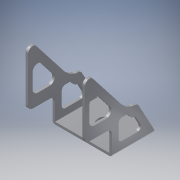
# Autodesk Inventor part: 頭_メインフレーム_1_1
Saved by Autodesk Inventor 2018 (Build 220112000, 112)
## iProperties
Created: 2016-05-10
Part Number: 頭_メインフレーム_1_1
Material: アルミニウム 5052
Document SubType Name: シート メタル
Designer: hiroaki
Density: 2.68 g/cm^3
Sheet Metal Rule: Default_mm
Appearance: アルミニウム - フラット
Mass: 7.8172 g
Surface Area: 48.1184 cm^2
Volume: 2.91687 cm^3
Flat Pattern Width: 4.175 cm
Flat Pattern Length: 12.6574 cm
Flat Pattern Area: 52.8444 cm^2
Sheet Metal Width: 41.750 mm
Sheet Metal Length: 126.574 mm
Sheet Metal Area: 5284.444 mm^2
Author: hiroaki
Autodesk Inventor part; units mm, degrees
ref_plane "YZ Plane" through (0, 0, 0) normal (1, 0, 0) x (0, 1, 0)
ref_plane "XZ Plane" through (0, 0, 0) normal (0, 1, 0) x (-1, 0, 0)
ref_plane "XY Plane" through (0, 0, 0) normal (0, 0, 1) x (1, 0, 0)
sketch "スケッチ1" plane through (0, 0, 0) normal (0, 0, 1) x (1, 0, 0)
  circle A0 centre (0, 0) radius 11 construction
  circle A1 centre (0, 8.5) radius 1.35
  circle A2 centre (0, 0) radius 5.05
  circle A3 centre (-8.5, 0) radius 1.35
  circle A4 centre (0, -8.5) radius 1.35
  circle A5 centre (8.5, 0) radius 1.35
  line L0 (-16.25, 11) -> (-16.25, -30.75)
  line L1 (-16.25, -30.75) -> (16.25, -30.75)
  line L2 (16.25, -30.75) -> (16.25, 11)
  line L3 (16.25, 11) -> (-16.25, 11)
  line L4 (-13.5, -1) -> (13.5, -1) construction
  line L5 (13.5, -1) -> (13.5, -28) construction
  line L6 (13.5, -28) -> (-13.5, -28) construction
  line L7 (-13.5, -28) -> (-13.5, -1) construction
  circle A6 centre (-13.5, -1) radius 1.35 construction
  circle A7 centre (-13.5, -1) radius 2.75 construction
  circle A8 centre (-13.5, -28) radius 2.75 construction
  point P0 (0, 11)
  point P1 (0, -30.75)
  point P2 (0, -1)
  dimension "d0" = 22
  dimension "d1" = 10.1
  dimension "d2" = 8.5
  dimension "d3" = 2.7
  dimension "d6" = 360
  dimension "d8" = 32.5
  dimension "d9" = 27
  dimension "d10" = 1
  dimension "d11" = 2.7
  dimension "d40" = 41.75
  constraints: 16 end point, 9 centre point, 5 coincident, 4 perpendicular, 4 tangent, 4 vertical alignment, 3 midpoint, 3 parallel, 1 horizontal, 1 vertical, 9 other
  measures "d0" diameter of A0
  measures "d1" diameter of A2
  measures "d2" distance of point (0, 0) A1.centre
  measures "d3" diameter of A1
  measures "d8" distance between parallel lines of L2 L0
  measures "d9" distance of L4.start L4.end
  measures "d10" distance from line of point (0, 0) L4
  measures "d11" diameter of A6
  measures "d40" distance between parallel lines of L3 L1
extrude "押し出し1" add sketch "スケッチ1" along normal blind 1.5
sketch "スケッチ2" plane through (-16.25, -30.75, 1.5001) normal (-1, 0, 0) x (0, -1, 0)
  line L0 (-41.75, 0) -> (0, 0)
  line L1 (0, 0) -> (0, 45.9999)
  line L2 (0, 45.9999) -> (-41.75, 45.9999)
  line L3 (-41.75, 45.9999) -> (-41.75, 0)
  constraints: 6 end point, 1 horizontal, 1 perpendicular, 1 vertical
edge flange "フランジ1" height 47.5 angle 90 thickness 1.5 bend radius 0.0001 thickness toward (-1, 0, 0) relief straight relief width 1.5 relief depth 0.75 edges at (-16.25, -9.875, 1.5) wall of the first edge with corners at (-16.25, 11, 1.5001) (-16.25, -30.75, 1.5001) (-16.2501, -30.75, 47.5) (-16.2501, 11, 47.5)
bend "曲げ1"
corner "コーナー1"
sketch "スケッチ3" plane through (-17.75, -30.75, 47.5) normal (-1, 0, 0) x (0, 0, 1)
  line L0 (0, 41.75) -> (0, 0) projected
  line L1 (-45.9999, 41.75) -> (0, 41.75) projected
  line L2 (-2.75, 29.75) -> (-29.75, 29.75) construction
  line L3 (-29.75, 29.75) -> (-29.75, 2.75) construction
  line L4 (-29.75, 2.75) -> (-2.75, 2.75) construction
  line L5 (-2.75, 2.75) -> (-2.75, 29.75) construction
  line L6 (0, 0) -> (-45.9999, 0) construction
  circle A0 centre (-2.75, 29.75) radius 1.35
  circle A1 centre (-2.75, 2.75) radius 1.35
  circle A2 centre (-29.75, 2.75) radius 1.35
  circle A3 centre (-29.75, 29.75) radius 1.35
  circle A4 centre (-2.75, 2.75) radius 2.75 construction
  line L7 (-23.0232, 22.0826) -> (-1.0567, 4.9169)
  arc A5 (-2.75, 0) -> (-1.0567, 4.9169) centre (-2.75, 2.75) ccw
  line L8 (-2.75, 0) -> (-2.75, -11.4677)
  line L9 (-2.75, -11.4677) -> (6.4192, -11.4677)
  line L10 (6.4192, -11.4677) -> (6.4192, 48.6525)
  line L11 (6.4192, 48.6525) -> (-30.25, 50.6687)
  circle A6 centre (-29.75, 29.75) radius 2.75 construction
  circle A7 centre (-16.25, 30.75) radius 11 construction
  arc A8 (-27.2491, 30.8936) -> (-23.0232, 22.0826) centre (-16.25, 30.75) ccw
  line L12 (-5.4497, 3.2733) -> (-25.4861, 18.9308)
  arc A9 (-5.4497, 3.2733) -> (-5.5, 2.75) centre (-2.75, 2.75) ccw
  arc A10 (-25.75, 19.1418) -> (-25.4861, 18.9308) centre (-16.25, 30.75) ccw
  line L13 (-5.5, 2.75) -> (-25.75, 2.75)
  line L14 (-25.75, 2.75) -> (-25.75, 19.1418)
  arc A11 (-27.2491, 30.8936) -> (-28.4327, 32.164) centre (-29.75, 29.75) ccw
  line L15 (-28.4327, 32.164) -> (-45.9999, 41.75)
  line L16 (-45.9999, 41.75) -> (-30.25, 50.6687)
  point P0 (-47.5, 30.75)
  point P1 (-2.75, 16.25)
  point P2 (-16.25, 29.75)
  dimension "d24" = 27
  dimension "d30" = 2.7
  dimension "d44" = 12
  dimension "d45" = 1
  dimension "d46" = 22
  dimension "d50" = 4
  dimension "d52" = 4
  constraints: 28 end point, 11 centre point, 11 coincident, 10 point on circle, 5 tangent, 4 perpendicular, 3 concentric, 3 equal radius, 3 parallel, 2 horizontal, 2 midpoint, 2 vertical, 2 vertical alignment, 1 collinear, 6 other
  measures "d24" distance of L2.start L2.end
  measures "d30" diameter of A0
  measures "d44" distance between parallel lines of L1 L2
  measures "d45" distance from line of L2 A7.centre
  measures "d46" diameter of A7
  measures "d50" radial gap between concentric circles of A10 A8
  measures "d52" distance between parallel lines of L3 L14
extrude "押し出し2" cut sketch "スケッチ3" against normal blind 1.5 contours L1 L16 L11 L10 L9 L8 A5 L0 | L0 A5 L7 A8 A11 L15 L1 | A0 | A1 | A2 | A3 | A9 L13 L14 A10 L12
mirror "ミラー1" about plane through (0, 0, 0) normal (1, 0, 0) of "押し出し2", "フランジ1"
sketch "スケッチ5" plane through (-17.75, -30.75, 1.5001) normal (-1, 0, 0) x (0, 0, 1)
  circle A0 centre (16.25, 2.75) radius 1.35 projected
  line L0 (43.25, 0) -> (0, 0) projected
  line L1 (-3.1343, -10.7624) -> (13.5, -10.7624)
  line L2 (13.5, -10.7624) -> (13.5, 16.25)
  line L3 (13.5, 16.25) -> (-3.1343, 16.25)
  line L4 (-3.1343, 16.25) -> (-3.1343, -10.7624)
  circle A1 centre (16.25, 2.75) radius 2.75 construction
  point P0 (-1.5, 30.75)
  dimension "d47" = 13.5
  constraints: 8 end point, 2 parallel, 2 tangent, 1 centre point, 1 coincident, 1 horizontal, 1 perpendicular
  measures "d47" distance from line of A0.centre L3
extrude "押し出し4" cut sketch "スケッチ5" against normal blind 100 contours L4 L3 L2 L1
fillet "フィレット1" radius 3 6 edges at (17, 0.1436, 20.2509) (-17, 0.1436, 20.2509) (-17, -14.5, 15) (-17, -30.75, 15) (17.0001, -14.5, 15) (17, -30.75, 15)
sketch "スケッチ6" plane through (-17.75, -14.5, 1.5001) normal (-1, 0, 0) x (0, 0, 1)
  line L0 (17.2251, 16.1007) -> (0, 25.5) projected
  line L1 (0, 25.5) -> (0, 0) projected
  line L2 (0, 0) -> (10.5, 0) projected
  line L3 (20.2499, -13.5) -> (20.2499, 2.8918) projected
  circle A0 centre (16.2499, 13.5) radius 1.35 projected
  line L4 (4, 18.7605) -> (12.9229, 13.8915)
  line L5 (4, 18.7605) -> (4, 4)
  line L6 (4, 4) -> (16.2499, 4)
  line L7 (16.2499, 4) -> (16.2499, 10.15)
  arc A1 (12.9229, 13.8915) -> (16.2499, 10.15) centre (16.2499, 13.5) ccw
  point P0 (-1.5, 14.5)
  dimension "d53" = 2
  dimension "d54" = 4
  dimension "d56" = 4
  dimension "d57" = 4
  dimension "d58" = 4
  constraints: 8 end point, 2 perpendicular, 2 point on circle, 1 centre point, 1 coincident, 1 parallel, 1 vertical
  measures "d53" radial gap between concentric circles of A1 A0
  measures "d54" distance between parallel lines of L0 L4
  measures "d56" distance between parallel lines of L7 L3
  measures "d57" distance between parallel lines of L2 L6
  measures "d58" distance between parallel lines of L1 L5
extrude "押し出し5" cut sketch "スケッチ6" against normal blind 10 contours L4 A1 L7 L6 L5
fillet "フィレット2" radius 2 5 edges at (-17, 4.2605, 5.5001) (-17, -4.35, 17.75) (-17, -10.5, 17.75) (-17, -10.5, 5.5001) (-17, -0.6085, 14.423)
mirror "ミラー2" about plane through (0, 0, 0) normal (1, 0, 0) of "フィレット2", "押し出し5"
fillet "フィレット3" radius 3 8 edges at (-17, -11.6082, 21.75) (-17, -28, 21.75) (-17, -28, 42) (-17, -27.4767, 42.0503) (17, -28, 42) (17, -27.4767, 42.0503) (17, -11.6082, 21.75) (17, -28, 21.75)
sketch "スケッチ7" plane through (-17.75, -14.5, 1.5001) normal (-1, 0, 0) x (0, 0, 1)
  circle A0 centre (16.25, 13.5) radius 1.35 projected
  circle A1 centre (16.25, 13.5) radius 1.35
  circle A2 centre (16.2499, -13.5) radius 1.35 projected
  circle A3 centre (16.2499, -13.5) radius 1.35
  circle A4 centre (43.2499, -13.5) radius 1.35 projected
  circle A5 centre (43.2499, -13.5) radius 1.35
  point P0 (-1.5, 14.5)
  constraints: 3 centre point, 3 coincident
extrude "押し出し6" add sketch "スケッチ7" against normal up to surface (1.5 mm away)
sketch "スケッチ8" plane through (17.75, -14.5, 1.5001) normal (1, 0, 0) x (0, 0, -1)
  circle A0 centre (-16.2499, -13.5) radius 1.35 projected
  circle A1 centre (-16.2499, -13.5) radius 1.35
  circle A2 centre (-16.2499, 13.5) radius 1.35 projected
  circle A3 centre (-16.2499, 13.5) radius 1.35
  circle A4 centre (-43.2499, -13.5) radius 1.35 projected
  circle A5 centre (-43.2499, -13.5) radius 1.35
  point P0 (1.5, 14.5)
  constraints: 3 centre point, 3 coincident
extrude "押し出し7" add sketch "スケッチ8" against normal up to surface (1.5 mm away)
sketch "スケッチ9" plane through (0, 0, 0) normal (0, 0, -1) x (-1, 0, 0)
  circle A0 centre (0, -8.5) radius 1.35 projected
  circle A1 centre (0, -8.5) radius 1.35
  circle A2 centre (8.5, 0) radius 1.35 projected
  circle A3 centre (8.5, 0) radius 1.35
  circle A4 centre (0, 8.5) radius 1.35 projected
  circle A5 centre (0, 8.5) radius 1.35
  circle A6 centre (-8.5, 0) radius 1.35 projected
  circle A7 centre (-8.5, 0) radius 1.35
  point P0 (0, 0)
  constraints: 4 centre point, 4 coincident
extrude "押し出し8" add sketch "スケッチ9" against normal up to surface (1.5 mm away)
equation "\"d56\" = d55"
equation "\"d57\" = d54"
equation "\"d14\" = BendReliefWidth"
equation "\"d15\" = BendReliefDepth"
equation "\"d16\" = MinimumRemnant"
equation "\"d17\" = BendRadius"
equation "\"d21\" = CornerReliefSize"
equation "\"d22\" = GapSize"
equation "\"d23\" = JacobiRadiusSize"
equation "\"d63\" = Thickness"
equation "\"BendRadius\" = Thickness"
equation "\"BendReliefWidth\" = Thickness"
equation "\"BendReliefDepth\" = 0.5 * Thickness"
equation "\"CornerReliefSize\" = 4 * Thickness"
equation "\"MinimumRemnant\" = 2 * Thickness"
equation "\"TransitionRadius\" = BendRadius"
equation "\"JacobiRadiusSize\" = BendRadius"
equation "\"GapSize\" = Thickness"
equation "\"d55\" = d54"
equation "\"Thickness\" = 1.5"
